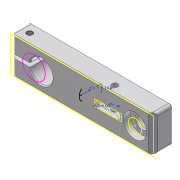
# Autodesk Inventor part: J002886
Saved by Autodesk Inventor 2012 SP2 (Build 160219200, 219)
## iProperties
Created: 2014-09-04
Material: ALUMINUM, 6061-T651
Vendor: HHMI: JFRC - ID&F
Document SubType Name: Modeling
Designer: arnoldj
Density: 2.7 g/cm^3
Mass: 2.44696 g
Surface Area: 8.61668 cm^2
Volume: 0.906283 cm^3
Part Number: J002886
Description: MPS Spring Mount
Project: P-194005
RuleStatus: InUse
AfterDocSave0: file://Part Number Cleaner
LAB/DEPT: SVOBODA (LAB)
REQUESTING SCIENTIST: PERON, SIMON
SURFACE ROUGHNESS: 63 Ra
DESIGN DEPARTMENT: HHMI: JFRC - ID&F
SPECIAL FINISH: ANODIZE PER MIL-A-8625F, TYPE II, CLASS 2 (BLACK)
ALTERED ITEM PART NUMBER: N/A
ALTERED ITEM VENDOR: N/A
ALTERED ITEM DESCRIPTION: N/A
Revision Number: -
Autodesk Inventor part; units mm, degrees
note: some values were not read from the file. Chosen so that the rebuilt part matches the saved one: direction of "Hole9".
ref_plane "YZ Plane" through (0, 0, 0) normal (1, 0, 0) x (0, 1, 0)
ref_plane "XZ Plane" through (0, 0, 0) normal (0, 1, 0) x (-1, 0, 0)
ref_plane "XY Plane" through (0, 0, 0) normal (0, 0, 1) x (1, 0, 0)
sketch "Sketch1" plane through (0, 0, 0) normal (0, 0, 1) x (1, 0, 0)
  line L0 (-19.05, 4.7625) -> (19.05, 4.7625)
  line L1 (19.05, 4.7625) -> (19.05, -4.7625)
  line L2 (19.05, -4.7625) -> (-19.05, -4.7625)
  line L3 (-19.05, -4.7625) -> (-19.05, 4.7625)
  point P0 (0, 0)
  point P1 (-19.05, 0)
  point P2 (0, 4.7625)
  dimension "d0" = 38.1
  dimension "d1" = 9.525
  constraints: 8 end point, 2 midpoint, 2 parallel, 1 horizontal, 1 horizontal alignment, 1 perpendicular, 1 vertical alignment
  measures "d0" distance of L0.start L0.end
  measures "d1" distance of L2.end L0.start
extrude "Extrusion1" add sketch "Sketch1" along normal blind 5.207
sketch "Sketch2" plane through (0, 0, 5.207) normal (0, 0, 1) x (1, 0, 0)
  line L0 (-19.05, -4.7625) -> (-19.05, 4.7625) projected
  point P0 (0, 0)
  point P1 (-10.795, 0)
  dimension "d4" = 8.255
  measures "d4" distance from line of L0 point (-10.795, 0)
hole "Hole1" at (-10.795, 0, 5.207) direction (0, 0, -1) diameter 6.0071 end through all
sketch "Sketch4" plane through (0, 0, 0) normal (1, 0, 0) x (0, 1, 0)
  circle A0 centre (0, 4.1099) radius 1.778
  point P0 (0, 0)
  dimension "d18" = 3.556
  constraints: 1 centre point
  measures "d18" diameter of A0
sketch "Sketch8" plane through (0, 0, 0) normal (0, 0, -1) x (-1, 0, 0)
  circle A0 centre (10.795, 0) radius 3.0035 projected
  circle A1 centre (10.795, 0) radius 4.7625 construction
  circle A2 centre (10.795, 0) radius 3.1115
  line L0 (-19.05, 4.7625) -> (-19.05, -4.7625) projected
  line L1 (19.05, 4.7625) -> (-19.05, 4.7625) projected
  line L2 (-19.05, -4.7625) -> (19.05, -4.7625) projected
  line L3 (19.05, -4.7625) -> (19.05, 4.7625) projected
  line L4 (-19.05, 4.7625) -> (19.05, 4.7625)
  line L5 (19.05, 4.7625) -> (19.05, -4.7625)
  line L6 (19.05, -4.7625) -> (-19.05, -4.7625)
  line L7 (-19.05, -4.7625) -> (-19.05, 4.7625)
  point P0 (17.78, -4.7625)
  point P1 (17.78, 4.7625)
  point P2 (0, 0)
  dimension "d52" = 9.525
  dimension "d53" = 6.223
  constraints: 8 end point, 2 centre point, 2 coincident, 2 parallel, 1 horizontal, 1 perpendicular
  measures "d52" diameter of A1
  measures "d53" diameter of A2
extrude "Extrusion4" [suppressed]
sketch "Sketch9" plane through (0, 0, 0) normal (0, 0, 1) x (1, 0, 0)
  line L0 (3.429, 0.889) -> (10.541, 0.889)
  line L1 (10.541, 0.889) -> (10.541, -0.889)
  line L2 (10.541, -0.889) -> (3.429, -0.889)
  line L3 (3.429, -0.889) -> (3.429, 0.889)
  line L4 (10.541, 0) -> (3.429, 0) construction
  line L5 (6.985, 0.889) -> (6.985, -0.889) construction
  circle A0 centre (-10.795, 0) radius 3.0035 projected
  point P0 (0, 0)
  dimension "d60" = 7.112
  dimension "d61" = 1.778
  dimension "d130" = 17.78
  constraints: 12 end point, 4 midpoint, 2 parallel, 1 horizontal, 1 horizontal alignment, 1 perpendicular
  measures "d60" distance of L0.start L0.end
  measures "d61" distance of L2.end L0.start
  measures "d130" distance from line of L5 A0.centre
extrude "Extrusion5" cut sketch "Sketch9" along normal up to next contours L0 L1 L2 L3
sketch "Sketch11" plane through (0, 0, 0) normal (0, 0, 1) x (1, 0, 0)
  line L0 (-26.67, 0) -> (26.67, 0) projected
  circle A0 centre (-10.795, 0) radius 3.0035 projected
  point P0 (0, 0)
  point P1 (14.224, 0)
  dimension "d131" = 25.019
  constraints: 1 point on line
  measures "d131" distance of point (14.224, 0) A0.centre
hole "Hole5" at (14.224, 0, 0) direction (0, 0, 1) diameter 3.5687 end through all counterbore diameter 6.0071 counterbore depth 2.667
sketch "Sketch13" plane through (0, 0, 0) normal (0, 1, 0) x (-1, 0, 0)
  line L0 (-10.541, 0) -> (-10.541, 5.207) projected
  line L1 (-3.429, 0) -> (-3.429, 5.207) projected
  line L2 (-10.541, 5.207) -> (-3.429, 5.207) construction
  line L3 (-6.985, 5.207) -> (-6.985, 3.302) construction
  point P0 (0, 0)
  point P1 (-8.89, 0.381)
  point P2 (-1.27, 0.381)
  dimension "d98" = 1.905
  constraints: 4 end point, 1 coincident, 1 horizontal, 1 midpoint, 1 perpendicular, 2 other
  measures "d98" distance of L3.start L3.end
hole "Hole6" at (6.985, 0, 3.302) direction (0, -1, 0) diameter 1.6256 end through all
hole "Hole7" at (6.985, 0, 3.302) direction (0, 1, 0) diameter 1.5748 end through all
sketch "Sketch18" plane through (0, 0, 5.207) normal (0, 0, 1) x (1, 0, 0)
  circle A0 centre (-10.795, 0) radius 3.0035 projected
  line L0 (-19.05, -4.7625) -> (-19.05, 4.7625) projected
  line L1 (-19.05, 0.508) -> (-13.7553, 0.508)
  line L2 (-13.7553, 0.508) -> (-13.7553, -0.508)
  line L3 (-13.7553, -0.508) -> (-19.05, -0.508)
  line L4 (-19.05, -0.508) -> (-19.05, 0.508)
  line L5 (-19.05, 0) -> (-13.7553, 0) construction
  point P0 (0, 0)
  point P1 (-19.05, 0)
  dimension "d132" = 1.016
  constraints: 10 end point, 3 midpoint, 2 parallel, 1 coincident, 1 horizontal, 1 perpendicular, 1 point on line, 2 other
  measures "d132" distance of L3.end L1.start
extrude "Extrusion7" cut sketch "Sketch18" against normal up to next contours L2 A0 | A0 L3 L0 L1 picked at (-13.7681, 0.0567)
sketch "Sketch19" plane through (-19.05, -4.7625, 0) normal (0, -1, 0) x (1, 0, 0)
  line L0 (38.1, 5.207) -> (0, 5.207) projected
  line L1 (0, 0) -> (0, 5.207) projected
  line L2 (5.2947, 0) -> (5.2947, 5.207) construction
  line L3 (0, 2.6035) -> (5.2947, 2.6035) construction
  line L4 (2.6474, 2.6035) -> (2.6474, 5.207) construction
  circle A0 centre (2.6474, 2.6035) radius 2.2225 construction
  point P0 (19.05, 0)
  dimension "d136" = 0
  dimension "d137" = 4.445
  constraints: 4 end point, 4 midpoint, 2 coincident, 1 centre point, 1 perpendicular, 1 point on line
  measures "d136" distance of L4.start point (2.647, 2.603)
  measures "d137" diameter of A0
hole "Hole9" at (-16.4026, -4.7625, 2.6035) direction (0, 1, 0) diameter 2.286 end up to surface counterbore diameter 4.445 counterbore depth 2.286
hole "Hole10" at (-16.4026, 0.508, 2.6035) direction (0, 1, 0) diameter 1.5748 end through all
sketch "Sketch20" plane through (0, 0, 5.207) normal (0, 0, 1) x (1, 0, 0)
  circle A0 centre (14.224, 0) radius 1.7844 projected
  point P0 (0, 0)
  constraints: 1 coincident
hole "Hole11" at (14.224, 0, 5.207) direction (0, 0, -1) diameter 6.223 depth 1.905
chamfer "Chamfer9" distance 1.27 angle 45 3 edges at (19.05, 0, 5.207) (-19.05, 2.6352, 5.207) (-19.05, -2.6353, 5.207)
sketch "Sketch15" plane through (0, 0, 0) normal (1, 0, 0) x (0, 1, 0)
  point P0 (0, 0)
sketch "Sketch16" plane through (0, 0, 5.207) normal (0, 0, 1) x (1, 0, 0)
  circle A0 centre (14.224, 0) radius 1.7844 projected
  line L0 (10.541, 0.889) -> (10.541, -0.889) projected
  line L1 (10.541, -0.889) -> (3.429, -0.889) projected
  line L2 (3.429, -0.889) -> (3.429, 0.889) projected
  line L3 (3.429, 0.889) -> (10.541, 0.889) projected
  circle A1 centre (-12.7, 0) radius 3.0035 projected
  line L4 (19.05, 4.7625) -> (19.05, -4.7625) projected
  line L5 (-19.05, 4.7625) -> (19.05, 4.7625) projected
  line L6 (-19.05, -4.7625) -> (-19.05, 4.7625) projected
  line L7 (19.05, -4.7625) -> (-19.05, -4.7625) projected
  point P0 (0, 0)
sketch "Sketch14" plane through (0, 0, 5.207) normal (0, 0, 1) x (1, 0, 0)
  circle A0 centre (6.985, 0) radius 4.1275
  line L0 (10.541, 0.889) -> (10.541, -0.889) projected
  line L1 (10.541, -0.889) -> (3.429, -0.889) projected
  line L2 (3.429, -0.889) -> (3.429, 0.889) projected
  line L3 (3.429, 0.889) -> (10.541, 0.889) projected
  line L4 (-17.78, 4.7625) -> (17.78, 4.7625) projected
  line L5 (17.78, -4.7625) -> (-17.78, -4.7625) projected
  line L6 (6.1976, 0.889) -> (6.1976, 4.7625) projected
  line L7 (7.7724, 0.889) -> (7.7724, 4.7625) projected
  line L8 (6.1976, 4.7625) -> (7.7724, 4.7625) construction
  line L9 (6.985, 4.7625) -> (6.985, -4.7625) construction
  line L10 (-13.7553, -0.508) -> (-17.78, -0.508) projected
  line L11 (-17.78, 0.508) -> (-13.7553, 0.508) projected
  arc A1 (-13.7553, -0.508) -> (-13.7553, 0.508) centre (-10.795, 0) ccw projected
  line L12 (17.78, 4.7625) -> (17.78, -4.7625) projected
  line L13 (-17.78, -4.7625) -> (-17.78, -0.508) projected
  line L14 (-17.78, 0.508) -> (-17.78, 4.7625) projected
  point P0 (0, 0)
  dimension "d113" = 8.255
  constraints: 4 end point, 2 midpoint, 2 perpendicular, 1 centre point, 1 coincident, 1 point on line
  measures "d113" diameter of A0
extrude "Extrusion6" [suppressed]
fillet "Fillet4" radius 0.889 4 edges at (10.541, 0.889, 2.6035) (10.541, -0.889, 2.6035) (3.429, 0.889, 2.6035) (3.429, -0.889, 2.6035)
fillet "Fillet5" radius 0.762 4 edges at (-19.05, 4.7625, 1.9685) (-19.05, -4.7625, 1.9685) (19.05, 4.7625, 1.9685) (19.05, -4.7625, 1.9685)
chamfer "Chamfer5" distance 0.254 angle 45 11 edges at (0, 4.7625, 5.207) (0, -4.7625, 5.207) (-19.05, -2.2543, 0) (-18.8268, -4.5393, 0) (0, -4.7625, 0) (18.8268, -4.5393, 0) (19.05, 0, 0) (18.8268, 4.5393, 0) (0, 4.7625, 0) (-18.8268, 4.5393, 0) (-19.05, 2.2542, 0)
sketch "Sketch12" plane through (0, 0, 0) normal (0, 1, 0) x (-1, 0, 0)
  point P0 (0, 0)
chamfer "Chamfer8" distance 0.254 angle 45 3 edges at (-7.7914, 0, 0) (14.224, -3.0035, 0) (-7.7914, 0, 5.207)
body "Solid1"
